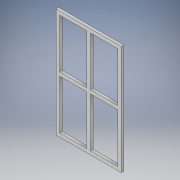
# Autodesk Inventor part: Door
Saved by Autodesk Inventor 2017 (Build 210142000, 142)
## iProperties
Created: 2016-09-12
Part Number: Door
Material: Generic
Document SubType Name: Modeling
Designer: s.ethan.wierenga
Density: 1 g/cm^3
Appearance: Default
Author: s.ethan.wierenga
Autodesk Inventor part; units mm, degrees
ref_plane "YZ Plane" through (0, 0, 0) normal (1, 0, 0) x (0, 1, 0)
ref_plane "XZ Plane" through (0, 0, 0) normal (0, 1, 0) x (-1, 0, 0)
ref_plane "XY Plane" through (0, 0, 0) normal (0, 0, 1) x (1, 0, 0)
sketch "Sketch1" plane through (0, 0, 0) normal (0, 0, 1) x (1, 0, 0)
  line L0 (0, 0) -> (466.725, 0)
  line L1 (466.725, 0) -> (466.725, 781.05)
  line L2 (466.725, 781.05) -> (0, 781.05)
  line L3 (0, 781.05) -> (0, 0)
  dimension "d0" = 466.725
  dimension "d1" = 781.05
  constraints: 8 end point, 2 parallel, 1 horizontal, 1 perpendicular
  measures "d0" distance of L2.end L1.end
  measures "d1" distance of L0.end L1.end
extrude "Extrusion1" add sketch "Sketch1" along normal blind 19.05
sketch "Sketch2" plane through (0, 0, 19.05) normal (0, 0, 1) x (1, 0, 0)
  line L0 (0, 0) -> (466.725, 0) projected
  line L1 (466.725, 0) -> (466.725, 781.05) projected
  line L2 (466.725, 781.05) -> (0, 781.05) projected
  line L3 (0, 781.05) -> (0, 0) projected
  line L4 (25.4, 755.65) -> (220.6625, 755.65)
  line L5 (220.6625, 755.65) -> (220.6625, 403.225)
  line L6 (220.6625, 403.225) -> (25.4, 403.225)
  line L7 (25.4, 403.225) -> (25.4, 755.65)
  line L8 (246.0625, 755.65) -> (441.325, 755.65)
  line L9 (441.325, 755.65) -> (441.325, 403.225)
  line L10 (441.325, 403.225) -> (246.0625, 403.225)
  line L11 (246.0625, 403.225) -> (246.0625, 755.65)
  line L12 (25.4, 377.825) -> (220.6625, 377.825)
  line L13 (220.6625, 377.825) -> (220.6625, 25.4)
  line L14 (220.6625, 25.4) -> (25.4, 25.4)
  line L15 (25.4, 25.4) -> (25.4, 377.825)
  line L16 (246.0625, 377.825) -> (441.325, 377.825)
  line L17 (441.325, 377.825) -> (441.325, 25.4)
  line L18 (441.325, 25.4) -> (246.0625, 25.4)
  line L19 (246.0625, 25.4) -> (246.0625, 377.825)
  dimension "d4" = 466.725
  dimension "d5" = 781.05
  dimension "d6" = 195.2625
  dimension "d7" = 25.4
  dimension "d8" = 25.4
  dimension "d9" = 195.2625
  dimension "d10" = 25.4
  dimension "d11" = 25.4
  dimension "d12" = 25.4
  dimension "d13" = 25.4
  dimension "d14" = 25.4
  dimension "d15" = 195.2625
  dimension "d16" = 25.4
  dimension "d17" = 195.2625
  dimension "d18" = 25.4
  dimension "d20" = 352.425
  dimension "d21" = 352.425
  constraints: 32 end point, 8 parallel, 4 horizontal, 4 perpendicular, 4 point on line
  measures "d4" distance between parallel lines of L1 L3
  measures "d5" distance of L0.end L1.end
  measures "d6" distance of L4.start L4.end
  measures "d7" distance between parallel lines of L7 L3
  measures "d8" distance between parallel lines of L11 L5
  measures "d9" distance of L8.start L8.end
  measures "d10" distance between parallel lines of L2 L8
  measures "d11" distance between parallel lines of L2 L4
  measures "d12" distance between parallel lines of L12 L6
  measures "d13" distance between parallel lines of L10 L16
  measures "d14" distance between parallel lines of L3 L15
  measures "d15" distance of L13.end L14.end
  measures "d16" distance between parallel lines of L1 L17
  measures "d17" distance of L17.end L18.end
  measures "d18" distance between parallel lines of L0 L14
  measures "d20" distance of L6.end L4.start
  measures "d21" distance of L14.end L12.start
extrude "Extrusion2" cut sketch "Sketch2" against normal blind 19.05 contours L4 L5 L6 L7 | L8 L9 L10 L11 | L12 L13 L14 L15 | L16 L17 L18 L19
body "Solid1"
